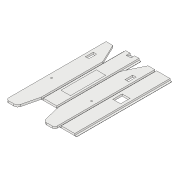
# Autodesk Inventor part: PF-01-0-0
Saved by Autodesk Inventor 2019 (Build 230136000, 136)
## iProperties
Created: 2022-03-20
Part Number: PF-01-0-0
Material: Foam board
Document SubType Name: Modeling
Designer: solyo
Density: 0.096049 g/cm^3
Appearance: Foam
Mass: 16.1334 g
Surface Area: 900.201 cm^2
Volume: 167.971 cm^3
Author: solyo
Autodesk Inventor part; units mm, degrees
ref_plane "YZ Plane" through (0, 0, 0) normal (1, 0, 0) x (0, 1, 0)
ref_plane "XZ Plane" through (0, 0, 0) normal (0, 1, 0) x (-1, 0, 0)
ref_plane "XY Plane" through (0, 0, 0) normal (0, 0, 1) x (1, 0, 0)
sketch "Sketch1" plane through (0, 0, 0) normal (0, 1, 0) x (-1, 0, 0)
  line L0 (168, 0) -> (168, 255)
  line L1 (168, 255) -> (140, 255)
  line L2 (140, 255) -> (128, 205)
  line L3 (0, 0) -> (0, 0) construction
  line L4 (0, 0) -> (39, 0) construction
  line L5 (72, 255) -> (84, 205)
  line L6 (128, 205) -> (128, 205)
  line L7 (128, 205) -> (84, 205)
  line L8 (84, 205) -> (84, 205)
  line L9 (106, 205) -> (106, 0) construction
  line L10 (72, 255) -> (44, 255)
  line L11 (44, 255) -> (44, 243)
  line L12 (44, 243) -> (0, 243)
  line L13 (0, 0) -> (61, 0)
  line L14 (22, 243) -> (22, -153.1158) construction
  line L15 (0, 243) -> (0, 0)
  line L16 (61, 0) -> (84, 48)
  line L17 (128, 48) -> (151, 0)
  line L18 (151, 0) -> (168, 0)
  line L19 (84, 48) -> (84, -5)
  line L20 (84, -5) -> (128, -5)
  line L21 (128, -5) -> (128, 48)
  point P0 (106, 48)
  point P1 (106, -5)
  dimension "d20" = 40
  dimension "d55" = 28
  dimension "d56" = 50
  dimension "d62" = 44
  dimension "d78" = 12
  dimension "d90" = 44
  dimension "d91" = 40
  dimension "d110" = 17
  dimension "d111" = 17
  dimension "d112" = 255
  dimension "d119" = 48
  dimension "d151" = 53
  constraints: 44 end point, 9 vertical, 5 horizontal alignment, 4 perpendicular, 3 horizontal, 3 midpoint, 2 point on line, 2 vertical alignment, 1 coincident, 1 collinear
  measures "d20" distance from line of L2.end L0
  measures "d55" distance of L0.end L1.end
  measures "d56" distance from line of L1 L2.end
  measures "d62" distance of L6.end L7.end
  measures "d78" distance between parallel lines of L10 L12
  measures "d90" distance of L11.end L12.end
  measures "d91" distance between parallel lines of L11 L8
  measures "d110" horizontal distance of L11.end L13.end
  measures "d111" distance of L17.end L0.start
  measures "d112" distance between parallel lines of L1 L18
  measures "d119" vertical distance of L0.start L17.start
  measures "d151" distance from line of L17.start L20
extrude "Extrusion1" add sketch "Sketch1" along normal blind 5
sketch "Sketch8" plane through (0, 5, 0) normal (0, 1, 0) x (1, 0, 0)
  line L0 (-32, -119) -> (-12, -119)
  line L1 (-12, -119) -> (-12, -95)
  line L2 (-12, -95) -> (-32, -95)
  line L3 (-32, -95) -> (-32, -119)
  line L4 (-44, -243) -> (0, -243) projected
  line L5 (-118, -165) -> (-94, -165)
  line L6 (-94, -165) -> (-94, -75)
  line L7 (-94, -75) -> (-118, -75)
  line L8 (-118, -75) -> (-118, -165)
  line L9 (-128, 5) -> (-128, -48) projected
  line L10 (-84, -48) -> (-84, 5) projected
  line L11 (-128, -205) -> (-84, -205) projected
  line L12 (-84, 5) -> (-128, 5) projected
  line L13 (-84, -205) -> (-72, -255) projected
  line L14 (-72, -255) -> (-44, -255) projected
  line L15 (-44, -255) -> (-44, -243) projected
  line L16 (-44, -243) -> (0, -243) projected
  line L17 (0, -243) -> (0, 0) projected
  line L18 (0, 0) -> (-61, 0) projected
  line L19 (-61, 0) -> (-84, -48) projected
  line L20 (-84, -48) -> (-84, 5) projected
  line L21 (-84, 5) -> (-128, 5) projected
  line L22 (-128, 5) -> (-128, -48) projected
  line L23 (-128, -48) -> (-151, 0) projected
  line L24 (-151, 0) -> (-168, 0) projected
  line L25 (-168, 0) -> (-168, -255) projected
  line L26 (-168, -255) -> (-140, -255) projected
  line L27 (-140, -255) -> (-128, -205) projected
  line L28 (-128, -205) -> (-84, -205) projected
  line L29 (-161, -40) -> (-161, -60)
  line L30 (-161, -60) -> (-152, -60)
  line L31 (-152, -60) -> (-152, -40)
  line L32 (0, 0) -> (-61, 0) projected
  line L33 (-60, -40) -> (-60, -60)
  line L34 (-60, -60) -> (-51, -60)
  line L35 (-51, -60) -> (-51, -40)
  line L36 (-161, -40) -> (-152, -40)
  line L37 (-60, -40) -> (-51, -40)
  point P0 (-22, -119)
  point P1 (-22, -243)
  dimension "d138" = 95
  dimension "d140" = 10
  dimension "d141" = 10
  dimension "d143" = 80
  dimension "d148" = 24
  dimension "d149" = 20
  dimension "d164" = 40
  dimension "d165" = 9
  dimension "d167" = 20
  dimension "d168" = 40
  dimension "d169" = 7
  dimension "d170" = 9
  dimension "d171" = 7
  constraints: 32 end point, 6 perpendicular, 4 parallel, 3 horizontal, 3 vertical, 2 collinear, 2 midpoint, 1 vertical alignment
  measures "d138" distance from line of L32.start L2
  measures "d140" distance between parallel lines of L9 L8
  measures "d141" distance between parallel lines of L10 L6
  measures "d143" distance between parallel lines of L12 L7
  measures "d148" distance of L2.end L0.start
  measures "d149" distance of L0.start L0.end
  measures "d164" distance between parallel lines of L11 L5
  measures "d165" distance of L33.end L34.end
  measures "d167" distance of L30.end L31.end
  measures "d168" distance between parallel lines of L24 L36
  measures "d169" distance between parallel lines of L25 L29
  measures "d170" distance of L29.start L31.end
  measures "d171" distance between parallel lines of L15 L35
extrude "Extrusion6" cut sketch "Sketch8" against normal through all contours L3 L2 L1 L0 | L36 L31 L30 L29 | L37 L35 L34 L33
sketch "Sketch4" plane through (0, 5, 0) normal (0, 1, 0) x (1, 0, 0)
  line L0 (-84, -205) -> (-72, -255) projected
  line L1 (-168, 0) -> (-168, -255) projected
  line L2 (-168, -255) -> (-140, -255) projected
  line L3 (-140, -255) -> (-128, -205) projected
  line L4 (-128, -205) -> (-84, -205) projected
  line L5 (-72, -255) -> (-44, -255) projected
  line L6 (-44, -255) -> (-44, -243) projected
  line L7 (-44, -243) -> (0, -243) projected
  line L8 (0, 0) -> (-61, 0) projected
  line L9 (0, -243) -> (0, 0) projected
  line L10 (-44, -243) -> (-44, 0)
  line L11 (-5, 0) -> (-5, -243)
  line L12 (-39, -243) -> (-39, 0)
  line L13 (-61, 0) -> (-84, -48) projected
  line L14 (-128, -48) -> (-151, 0) projected
  line L15 (-151, 0) -> (-168, 0) projected
  line L16 (-128, -205) -> (-128, -48)
  line L17 (-84, -205) -> (-84, -48)
  line L18 (-84, -48) -> (-84, 5) projected
  line L19 (-84, 5) -> (-128, 5) projected
  line L20 (-128, 5) -> (-128, -48) projected
  line L21 (-123, -205) -> (-123, 5)
  line L22 (-89, 5) -> (-89, -205)
  dimension "d97" = 5
  dimension "d98" = 5
  dimension "d156" = 5
  dimension "d157" = 5
  constraints: 14 end point, 9 point on line, 4 vertical, 1 parallel, 1 perpendicular
  measures "d97" distance between parallel lines of L10 L12
  measures "d98" distance between parallel lines of L9 L11
  measures "d156" distance between parallel lines of L16 L21
  measures "d157" distance between parallel lines of L17 L22
extrude "Extrusion4" cut sketch "Sketch4" against normal blind 4.5 contours L4 L22 L19 L18 L17 | L4 L16 L20 L19 L21 | L10 L8 L12 L7 | L11 L8 L9 L7
ref_plane "Work Plane11" through (-106, 5, 205) normal (1, 0, 0) x (0, 0, -1)
sketch "Sketch9" plane through (-106, 5, 205) normal (1, 0, 0) x (0, 0, -1)
  line L0 (210, -4.5) -> (210, 0) projected
  line L1 (210, 0) -> (0, 0) projected
  line L2 (157, -4.5) -> (210, -4.5) projected
  line L3 (210, -4.5) -> (200.3497, 0)
  point P0 (205, -5)
  point P1 (146, -4.5)
  dimension "d158" = 65
  constraints: 2 end point, 1 point on line
  measures "d158" angle of L3 L0
extrude "Extrusion7" cut sketch "Sketch9" along normal mid plane 12
split body "Split13" sketch "Sketch8" result two bodies curves L7 L8 L5 L6 first body at (-110, 0.5, 105)
sketch "Sketch7" plane through (0, 5, 0) normal (0, 1, 0) x (1, 0, 0)
  line L0 (-168, 0) -> (-168, -255) projected
  line L1 (-44, -255) -> (-44, 0) projected
  line L2 (-168, -255) -> (-140, -255) projected
  line L3 (-151, 0) -> (-168, 0) projected
  point P0 (0, 0)
  point P1 (-55, -150)
  point P2 (-157, -150)
  dimension "d120" = 11
  dimension "d121" = 11
  dimension "d172" = 150
  constraints: 1 horizontal alignment
  measures "d120" distance from line of point (-157, -150) L0
  measures "d121" distance from line of L1 point (-55, -150)
  measures "d172" distance from line of L3 point (-157, -150)
hole "Hole1" at (-55, 5, 150) at (-157, 5, 150) direction (0, -1, 0) diameter 4 end through all bodies 2 3
fillet "Fillet1" radius 10 2 edges at (-140, 2.5, 255) (-72, 2.5, 255)
fillet "Fillet1" radius 6 2 edges at (-44, 2.5, 255) (-168, 2.5, 255)
equation "\"d35\" = Thickness"
equation "\"Thickness\" = 5"
equation "\"Paper\" = 0.5"
equation "\"Camber\" = 34"
body "Solid28"
body "Solid29"
body "Solid30"
body "Solid31"
body "Solid32"
body "Solid33"
body "Solid34"
body "Solid35"
body "Solid36"
body "Solid37"
